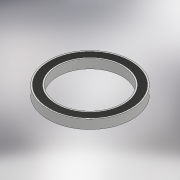
# Autodesk Inventor part: 65x50x7 bearing
Saved by Autodesk Inventor 2020.3 (Build 243373000, 373)
## iProperties
Created: 2018-05-07
Part Number: 65x50x7 bearing
Material: Generic
Document SubType Name: Modeling
Designer: paulg
Density: 5.72292 g/cm^3
Appearance: Default
Mass: 52 g
Surface Area: 53.8312 cm^2
Volume: 9.08627 cm^3
Author: paulg
Autodesk Inventor part; units mm, degrees
ref_plane "YZ Plane" through (0, 0, 0) normal (1, 0, 0) x (0, 1, 0)
ref_plane "XZ Plane" through (0, 0, 0) normal (0, 1, 0) x (-1, 0, 0)
sketch "Sketch1" plane through (0, 0, 0) normal (0, 0, 1) x (1, 0, 0)
  circle A0 centre (0, 0) radius 32.5
  circle A1 centre (0, 0) radius 25
  circle A2 centre (0, 0) radius 26
  circle A3 centre (0, 0) radius 31.5
  dimension "d0" = 65
  dimension "d1" = 50
  dimension "d2" = 1
  dimension "d3" = 1
  constraints: 4 centre point, 4 coincident
  measures "d0" diameter of A0
  measures "d1" diameter of A1
  measures "d2" radial gap between concentric circles of A1 A2
  measures "d3" radial gap between concentric circles of A0 A3
extrude "Extrusion1" add sketch "Sketch1" along normal blind 7
ref_plane "Work Plane1" through (0, 0, 0.2) normal (0, 0, 1) x (1, 0, 0)
sketch "Sketch2" plane through (0, 0, 0.2) normal (0, 0, 1) x (1, 0, 0)
  circle A0 centre (0, 0) radius 31.5 projected
  circle A1 centre (0, 0) radius 32.5 projected
  circle A2 centre (0, 0) radius 25 projected
  circle A3 centre (0, 0) radius 26 projected
extrude "Extrusion2" add sketch "Sketch2" along normal blind 6.6 contours A0
body "Solid1"
